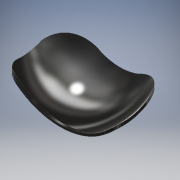
# Autodesk Inventor part: front
Saved by Autodesk Inventor 2017 (Build 210142000, 142)
## iProperties
Part Number: front
Material: Genérico
Document SubType Name: Modeling
Designer: Roberto
Density: 1 g/cm^3
Appearance: Valor por defecto
Author: Roberto
Autodesk Inventor part; units mm, degrees
ref_plane "XZ Plane" through (0, 0, 0) normal (0, 1, 0) x (-1, 0, 0)
ref_plane "XY Plane" through (0, 0, 0) normal (0, 0, 1) x (1, 0, 0)
sketch "Boceto1" plane through (0, 0, 0) normal (0, 0, 1) x (1, 0, 0)
  line L0 (-0.6113, 3.2908) -> (-0.374, 3.3479)
  line L1 (0.2767, 0) -> (-0.374, 3.3479)
  line L2 (-0.374, 3.3479) -> (0.2767, 0)
  line L3 (-0.6113, 3.2908) -> (0, 0)
  line L4 (-0.6113, 3.2908) -> (0, 0)
  line L5 (0, 0) -> (0.3056, 0)
  line L6 (0.2767, 0) -> (0, 0)
  line L7 (0, 0) -> (0.3056, 0)
  line L8 (0, 0) -> (15, 0)
  arc A0 (3.9618, 11.347) -> (-0.374, 3.3479) centre (7.6858, 4.1538) ccw
  arc A1 (7.5, 12.385) -> (3.8946, 11.3118) centre (8.3964, 2.7813) ccw
  line L9 (7.5, 12.6279) -> (7.5, 12.385)
  arc A2 (7.5, 12.6279) -> (3.8504, 11.5616) centre (8.3964, 2.7813) ccw
  arc A3 (3.8504, 11.5616) -> (-0.6113, 3.2908) centre (7.6858, 4.1538) ccw
  dimension "d0" = 15
  constraints: 20 end point, 11 point on circle, 4 centre point, 3 collinear, 3 horizontal, 2 coincident, 1 vertical
  measures "d0" distance of L5.start L8.end
revolve "Revolución1" add sketch "Boceto1" angle 180 about axis through (7.5, 12.6279, 0) along (0, -1, 0)
sketch "Boceto3" plane through (7.6858, 4.1538, 0) normal (0, 0, 1) x (0.8801, -0.4748, 0)
  line L0 (-4.5487, -7.1734) -> (8.1658, -0.3145) projected
  line L1 (2.4843, 0.0494) -> (0.3845, -1.1035)
  line L2 (-4.2082, -3.5805) -> (0.3845, -1.1035)
  line L3 (8.1661, -0.3151) -> (-4.549, -7.1729)
  line L4 (4.7704, 1.2824) -> (2.6706, 0.1295)
  arc A0 (4.7704, 1.2824) -> (5.1721, 2.7744) centre (4.255, 2.2212) ccw
  arc A1 (3.76, 5.1155) -> (-1.017, 5.8755) centre (0.9518, 2.8575) ccw
  line L5 (3.76, 5.1155) -> (5.1721, 2.7744)
  line L6 (-4.6978, 3.8903) -> (-1.017, 5.8755)
  line L7 (-2.9805, -2.9082) -> (3.7205, 0.706)
  line L8 (-1.922, -2.3475) -> (2.6706, 0.1295)
  arc A2 (-5.5062, -2.9849) -> (-4.0389, -3.4689) centre (-4.5402, -2.5225) ccw
  line L9 (-6.6869, -0.519) -> (-5.5062, -2.9849)
  arc A3 (-4.6978, 3.8903) -> (-6.6869, -0.519) centre (-3.2575, 0.5873) ccw
  line L10 (-4.7925, -7.3042) -> (-1.647, -5.6074)
  line L11 (1.8086, -3.744) -> (5.7443, -10.6485)
  line L12 (-4.0389, -3.4689) -> (4.7704, 1.2824)
  line L13 (-4.6978, 3.8903) -> (-1.017, 5.8755)
  line L14 (-5.5062, -2.9849) -> (-6.6869, -0.519)
  line L15 (5.1721, 2.7744) -> (3.76, 5.1155)
  point P0 (-4.7922, -7.3048)
  point P1 (-2.2994, -5.96)
  point P2 (5.9165, -1.5279)
  constraints: 30 end point, 8 point on circle, 4 centre point, 2 midpoint, 2 parallel, 1 collinear
extrude "Extrusión2" cut sketch "Boceto3" against normal blind 10 contours L12 A2 L9 A3 L6 A1 L5 A0 keep common part
ref_plane "Plano de trabajo1" through (7.5, 0, 0) normal (1, 0, 0) x (0, 1, 0)
